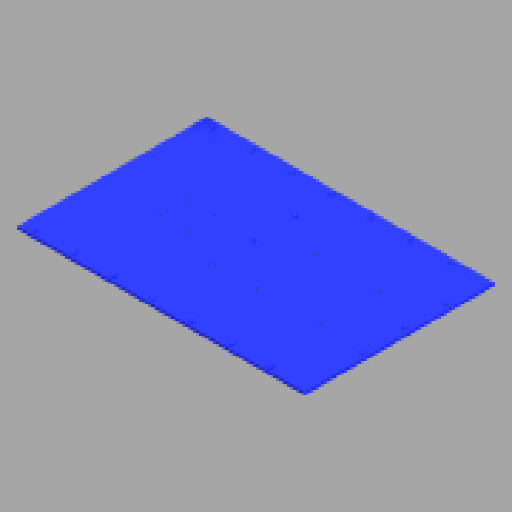
# Autodesk Inventor part: вверхняя плита
Saved by Autodesk Inventor 2025 (Build 290162000, 162)
## iProperties
Created: 2025-02-24
Part Number: вверхняя плита
Material: Алюминий 6061
Document SubType Name: Modeling
Designer: volko
Density: 2.7 g/cm^3
Appearance: Алюминий — плоский
Mass: 1927.01 g
Surface Area: 3672.19 cm^2
Volume: 713.709 cm^3
Author: volko
Autodesk Inventor part; units mm, degrees
ref_plane "YZ Plane" through (0, 0, 0) normal (1, 0, 0) x (0, 1, 0)
ref_plane "XZ Plane" through (0, 0, 0) normal (0, 1, 0) x (-1, 0, 0)
ref_plane "XY Plane" through (0, 0, 0) normal (0, 0, 1) x (1, 0, 0)
sketch "Эскиз1" plane through (0, 0, 0) normal (0, 1, 0) x (-1, 0, 0)
  line L0 (-265, 175) -> (-265, -175)
  line L1 (265, -175) -> (265, 175)
  line L2 (0, -245) -> (0, 245) projected
  line L3 (371, 0) -> (-371, 0) projected
  line L4 (265, 175) -> (-265, 175)
  line L5 (-125, 175) -> (-265, 175)
  line L6 (265, -175) -> (-265, -175)
  point P0 (0, 0)
  dimension "d0" = 530
  dimension "d1" = 350
  constraints: 10 end point, 3 horizontal, 2 perpendicular, 1 collinear, 1 parallel, 2 other
  measures "d0" distance of L0.start L1.end
  measures "d1" distance of L1.start L1.end
extrude "Выдавливание1" add sketch "Эскиз1" along normal blind 5
sketch "Эскиз2" plane through (0, 5, 0) normal (0, 1, 0) x (1, 0, 0)
  line L0 (0, 245) -> (0, -245) projected
  line L1 (-419, 0) -> (379, 0) projected
  line L2 (265, 175) -> (-265, 175) projected
  line L3 (265, -175) -> (265, 175) projected
  point P0 (0, 0)
  point P1 (0, 0)
  point P2 (255, 87.5)
  point P3 (0, 0)
  point P4 (255, 0)
  point P5 (255, -87.5)
  point P6 (0, 87.5)
  point P7 (0, 0)
  point P8 (0, -87.5)
  point P9 (-255, 87.5)
  point P10 (-255, 0)
  point P11 (-255, -87.5)
  point P12 (198.75, 165)
  point P13 (132.5, 165)
  point P14 (66.25, 165)
  point P15 (0, 165)
  point P16 (-66.25, 165)
  point P17 (-132.5, 165)
  point P18 (-198.75, 165)
  point P19 (198.75, -165)
  point P20 (132.5, -165)
  point P21 (66.25, -165)
  point P22 (0, -165)
  point P23 (-66.25, -165)
  point P24 (-132.5, -165)
  point P25 (-198.75, -165)
  dimension "d44" = 87.5
  dimension "d45" = 10
  dimension "d48" = 87.5
  dimension "d51" = 255
  dimension "d54" = 10
  dimension "d55" = 66.25
  dimension "d58" = 66.25
  dimension "d61" = 330
  constraints: 2 horizontal, 2 vertical, 1 coincident, 21 other
  measures "d44" distance from line of L2 point (255, 87.5)
  measures "d45" distance from line of L3 point (255, 87.5)
  measures "d48" distance of point (255, 87.5) point (255, 0)
  measures "d51" distance of point (255, 87.5) point (0, 87.5)
  measures "d54" distance from line of point (198.75, 165) L2
  measures "d55" distance from line of L3 point (198.75, 165)
  measures "d58" distance of point (198.75, 165) point (132.5, 165)
  measures "d61" distance of point (198.75, 165) point (198.75, -165)
hole "Отверстие1" at (-198.75, 5, 165) at (-132.5, 5, 165) at (-66.25, 5, 165) at (-198.75, 5, -165) at (-132.5, 5, -165) at (-66.25, 5, -165) at (-255, 5, 87.5) at (-255, 5, 0) at (-255, 5, -87.5) at (0, 5, 165) at (66.25, 5, 165) at (132.5, 5, 165) at (198.75, 5, 165) at (0, 5, -165) at (66.25, 5, -165) at (132.5, 5, -165) at (198.75, 5, -165) at (0, 5, 87.5) at (0, 5, 0) at (0, 5, -87.5) at (255, 5, 87.5) at (255, 5, 0) at (255, 5, -87.5) direction (0, -1, 0) diameter 5.5 end through all countersink diameter 11 countersink angle 90
sketch "Эскиз3" plane through (0, 5, 0) normal (0, 1, 0) x (1, 0, 0)
  line L0 (-371, 0) -> (371, 0) projected
  line L1 (0, 245) -> (0, -245) projected
  point P0 (0, 0)
  point P1 (-150, 25)
  point P2 (-100, 25)
  point P3 (-150, -25)
  point P4 (-100, -25)
  dimension "d73" = 50
  dimension "d76" = 50
  dimension "d79" = 100
  constraints: 1 horizontal, 1 symmetric about line, 1 vertical, 3 other
  measures "d73" distance of point (-150, 25) point (-100, 25)
  measures "d76" distance of point (-150, 25) point (-150, -25)
  measures "d79" distance from line of L1 point (-100, 25)
hole "Отверстие2" at (-150, 5, -25) at (-100, 5, 25) at (-100, 5, -25) at (-150, 5, 25) direction (0, -1, 0) diameter 4.134 end through all thread size "M5x0.8" class "6H" standard "ISO Metric profile"
sketch "Эскиз4" plane through (0, 5, 0) normal (0, 1, 0) x (1, 0, 0)
  line L0 (-371, 0) -> (371, 0) projected
  line L1 (-265, 175) -> (-265, -175) construction
  point P0 (0, 0)
  point P1 (-215, 23.4)
  point P2 (-215, -23.4)
  point P3 (-183.083, 0)
  dimension "d87" = 46.8
  dimension "d88" = 31.917
  dimension "d89" = 50
  constraints: 1 point on line, 1 symmetric about line
  measures "d87" distance of point (-215, -23.4) point (-215, 23.4)
  measures "d88" horizontal distance of point (-215, 23.4) point (-183.083, 0)
  measures "d89" distance from line of point (-215, 23.4) L1
hole "Отверстие3" at (-215, 5, -23.4) at (-183.083, 5, 0) at (-215, 5, 23.4) direction (0, -1, 0) diameter 1.567 end through all thread size "M2x0.4" class "6H" standard "ISO Metric profile"
sketch "Эскиз6" plane through (0, 5, 0) normal (0, 1, 0) x (1, 0, 0)
  line L0 (-371, 0) -> (371, 0) projected
  line L1 (0, 245) -> (0, -245) projected
  line L2 (265, -175) -> (265, 175) projected
  point P0 (0, 0)
  point P1 (175, 55)
  point P2 (56, 55)
  point P3 (175, -55)
  point P4 (56, -55)
  dimension "d109" = 119
  dimension "d112" = 110
  dimension "d115" = 90
  constraints: 1 horizontal, 1 symmetric about line, 1 vertical, 3 other
  measures "d109" distance of point (175, 55) point (56, 55)
  measures "d112" distance of point (175, 55) point (175, -55)
  measures "d115" distance from line of L2 point (175, 55)
hole "Отверстие5" at (175, 5, -55) at (56, 5, 55) at (175, 5, 55) at (56, 5, -55) direction (0, -1, 0) diameter 4.917 end through all thread size "M6x1" class "6H" standard "ISO Metric profile"
